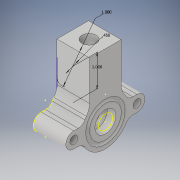
# Autodesk Inventor part: PeerIntput
Saved by Autodesk Inventor 2018 (Build 220112000, 112)
## iProperties
Created: 2020-03-28
Part Number: PeerIntput
Material: Generic
Document SubType Name: Modeling
Designer: emile
Density: 1 g/cm^3
Appearance: Default
Mass: 52.8326 g
Surface Area: 134.532 cm^2
Volume: 52.8326 cm^3
Author: emile
Title: T CROSSING INPUT TO MASK
Autodesk Inventor part; units mm, degrees
ref_plane "YZ Plane" through (0, 0, 0) normal (1, 0, 0) x (0, 1, 0)
ref_plane "XZ Plane" through (0, 0, 0) normal (0, 1, 0) x (-1, 0, 0)
ref_plane "XY Plane" through (0, 0, 0) normal (0, 0, 1) x (1, 0, 0)
sketch "Sketch2" plane through (0, 0, 0) normal (0, 0, 1) x (1, 0, 0)
  line L0 (-26.2255, 19.05) -> (26.2255, 19.05)
  line L1 (26.2255, 19.05) -> (26.2255, 0)
  line L2 (26.2255, 0) -> (-26.2255, 0)
  line L3 (-26.2255, 0) -> (-26.2255, 19.05)
  line L4 (-9.7155, 5.715) -> (-6.985, 8.4455)
  line L5 (-9.7155, 5.715) -> (-26.2255, 5.715)
  line L6 (-6.985, 8.4455) -> (0, 8.4455)
  line L7 (0, 8.4455) -> (0, 0)
  line L8 (0, 8.4455) -> (0, 19.05)
  line L9 (-3.9523, 10.7598) -> (-6.1075, 8.6046) construction
  circle A0 centre (0, 14.2875) radius 1.524
  dimension "d10" = 19.05
  dimension "d11" = 16.51
  dimension "d35" = 45
  dimension "d36" = 0.508
  dimension "d38" = 5.715
  dimension "d39" = 8.4455
  dimension "d40" = 3.048
  dimension "d41" = 14.2875
  dimension "d60" = 6.985
  constraints: 20 end point, 3 parallel, 3 perpendicular, 2 horizontal, 2 midpoint, 2 point on line, 1 centre point, 1 coincident
  measures "d10" distance between parallel lines of L2 L0
  measures "d11" distance from line of L3 L4.start
  measures "d35" angle of L6 L4
  measures "d36" distance between parallel lines of L4 L9
  measures "d38" distance between parallel lines of L2 L5
  measures "d39" distance between parallel lines of L2 L6
  measures "d40" diameter of A0
  measures "d41" distance from line of L2 A0.centre
  measures "d60" distance of L4.end L6.end
revolve "Revolution1" add sketch "Sketch2" angle 360 about axis through (26.2255, 0, 0) along (-1, 0, 0) picked at (-0.475, 14.1074) contours L0 L8 A0 L6 L4 L5 L3 | L8 A0
sketch "Sketch3" plane through (0, 0, 0) normal (1, 0, 0) x (0, 0, -1)
  circle A0 centre (-25.4, 0) radius 3.175
  line L0 (-25.4, -6.35) -> (-17.9605, -6.35)
  circle A1 centre (0, 0) radius 19.05 projected
  line L1 (-25.4, 6.35) -> (-17.9605, 6.35)
  arc A2 (-25.4, 6.35) -> (-25.4, -6.35) centre (-25.4, 0) ccw
  point P0 (0, 0)
  dimension "d20" = 6.35
  dimension "d21" = 25.4
  dimension "d22" = 12.7
  constraints: 4 end point, 4 point on circle, 2 centre point, 2 tangent, 1 coincident, 1 horizontal, 1 horizontal alignment, 1 parallel
  measures "d20" diameter of A0
  measures "d21" distance of point (0, 0) A0.centre
  measures "d22" distance between parallel lines of L0 L1
extrude "Extrusion2" add sketch "Sketch3" against normal up to surface (26.2255 mm away) contours A2 L1 A1 L0
fillet "Fillet1" radius 6.35 2 edges at (-13.1128, -6.35, 17.9605) (-13.1128, 6.35, 17.9605)
pattern_circular "Circular Pattern1" count 2 over 360 about axis through (-13.1127, 0, 0) along (1, 0, 0) of "Extrusion2", "Fillet1"
revolve "Revolution2" cut sketch "Sketch2" angle 360 about axis through (26.2255, 0, 0) along (-1, 0, 0) contours A0 L8 | L8 A0
sketch "Sketch10" plane through (-26.2255, 0, 25.4) normal (-1, 0, 0) x (0, 0, 1)
  arc A0 (-12.7, 25.4) -> (-38.1, 25.4) centre (-25.4, 25.4) ccw
  circle A1 centre (-50.8, 0) radius 3.175 projected
  circle A2 centre (0, 0) radius 3.175 projected
  circle A3 centre (-25.4, 0) radius 5.715 projected
  arc A4 (-3.403, -6.35) -> (-8.9022, -9.525) centre (-3.403, -12.7) ccw projected
  line L0 (0, -6.35) -> (-3.403, -6.35) projected
  arc A5 (0, -6.35) -> (0, 6.35) centre (0, 0) ccw projected
  line L1 (-3.403, 6.35) -> (0, 6.35) projected
  arc A6 (-8.9022, 9.525) -> (-3.403, 6.35) centre (-3.403, 12.7) ccw projected
  arc A7 (-8.9022, 9.525) -> (-41.8978, 9.525) centre (-25.4, 0) ccw projected
  arc A8 (-47.397, 6.35) -> (-41.8978, 9.525) centre (-47.397, 12.7) ccw projected
  line L2 (-50.8, 6.35) -> (-47.397, 6.35) projected
  arc A9 (-50.8, 6.35) -> (-50.8, -6.35) centre (-50.8, 0) ccw projected
  line L3 (-47.397, -6.35) -> (-50.8, -6.35) projected
  arc A10 (-41.8978, -9.525) -> (-47.397, -6.35) centre (-47.397, -12.7) ccw projected
  arc A11 (-41.8978, -9.525) -> (-8.9022, -9.525) centre (-25.4, 0) ccw projected
  line L4 (-38.1, 25.4) -> (-38.1, 14.199)
  line L5 (-12.7, 25.4) -> (-12.7, 14.199)
  circle A12 centre (-25.4, 25.4) radius 5.715
  line L6 (-12.7, 25.4) -> (-12.7, 38.1)
  line L7 (-12.7, 38.1) -> (-38.1, 38.1)
  line L8 (-38.1, 38.1) -> (-38.1, 25.4)
  point P0 (-25.4, 0)
  dimension "d61" = 25.4
  dimension "d62" = 11.43
  dimension "d63" = 25.4
  constraints: 10 end point, 4 point on circle, 4 tangent, 2 centre point, 2 perpendicular, 2 vertical, 1 coincident, 1 parallel, 1 vertical alignment
  measures "d61" diameter of A0
  measures "d62" diameter of A12
  measures "d63" distance of A3.centre A12.centre
extrude "Extrusion8" add sketch "Sketch10" against normal up to surface (26.2255 mm away) contours L5 A7 L4 A0 | A0 L7 L6 | A0 L8 L7 | A12
sketch "Sketch11" plane through (0, 0, 0) normal (1, 0, 0) x (0, 0, -1)
  circle A0 centre (0, 0) radius 5.715 projected
  point P0 (0, 0)
sketch "Sketch12" plane through (0, 0, 0) normal (0, 1, 0) x (-1, 0, 0)
  line L0 (0, 8.4455) -> (0, -8.4455) projected
  line L1 (6.985, 8.4455) -> (6.985, -8.4455) projected
  circle A0 centre (5.3975, 0) radius 1.5875
  circle A1 centre (5.3975, 5.08) radius 1.5875
  circle A2 centre (5.3975, -5.08) radius 1.5875
  point P0 (0, 0)
  dimension "d67" = 3.175
  dimension "d68" = 5.08
  dimension "d69" = 5.08
  dimension "d70" = 0
  constraints: 3 centre point, 2 equal radius, 1 horizontal alignment, 1 tangent, 1 vertical alignment
  measures "d67" diameter of A0
  measures "d68" distance of A1.centre A0.centre
  measures "d69" distance of A0.centre A2.centre
  measures "d70" horizontal distance of A0.centre A1.centre
extrude "Extrusion9" cut sketch "Sketch12" along normal blind 19.05
sketch "Sketch14" plane through (-5.3975, 19.05, 5.08) normal (0, -1, 0) x (1, 0, 0)
  point P0 (5.3975, -5.08)
sketch "Sketch15" plane through (-26.2255, 38.1, 12.7) normal (0, 1, 0) x (1, 0, 0)
  line L0 (26.2255, 0) -> (26.2255, 25.4) projected
  line L1 (0, 25.4) -> (26.2255, 25.4) projected
  line L2 (0, 0) -> (0, 25.4) projected
  line L3 (0, 0) -> (26.2255, 0) projected
  circle A0 centre (13.1128, 12.7) radius 5.715
  line L4 (26.2255, 0) -> (26.2255, 25.4) projected
  point P0 (26.2255, 12.7)
  point P1 (26.2255, 12.7)
  point P2 (13.1128, 0)
  dimension "d75" = 11.43
  constraints: 2 midpoint, 1 centre point, 1 horizontal alignment, 1 vertical alignment
  measures "d75" diameter of A0
loft "Loft1" cut profiles "Sketch15" section 1 edges at (-3.81, 19.05, 5.08) contours A0
loft "Loft2" cut section 1 edges at (-13.1128, 38.1, 5.715) (-13.1128, 38.1, -5.715) section 2 edges at (-3.81, 19.05, 0)
loft "Loft3" cut section 1 edges at (-13.1128, 38.1, -5.715) (-13.1128, 38.1, 5.715) section 2 edges at (-3.81, 19.05, -5.08)
sketch "Sketch16" plane through (-26.2255, 38.1, 12.7) normal (0, 1, 0) x (1, 0, 0)
  arc A0 (18.8278, 12.7) -> (7.3978, 12.7) centre (13.1128, 12.7) ccw projected
  arc A1 (7.3978, 12.7) -> (18.8278, 12.7) centre (13.1128, 12.7) ccw projected
  line L0 (26.2255, 0) -> (26.2255, 25.4) projected
  line L1 (0, 25.4) -> (26.2255, 25.4) projected
  line L2 (0, 0) -> (0, 25.4) projected
  line L3 (0, 0) -> (26.2255, 0) projected
  point P0 (26.2255, 12.7)
extrude "Extrusion11" add sketch "Sketch16" along normal blind 12.7
fillet "Fillet4" radius 12.7 2 edges at (-13.1128, 14.199, -12.7) (-13.1128, 14.199, 12.7)
equation "\"d69\" = d68"
body "Solid2"
